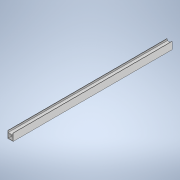
# Autodesk Inventor part: rail
Saved by Autodesk Inventor 2021 (Build 250183000, 183)
## iProperties
Created: 2021-04-01
Part Number: rail
Material: Generic
Document SubType Name: Modeling
Designer: miw14
Density: 1 g/cm^3
Appearance: Default
Mass: 103313 g
Surface Area: 104654 cm^2
Volume: 103313 cm^3
Author: miw14
Autodesk Inventor part; units mm, degrees
ref_plane "YZ Plane" through (0, 0, 0) normal (1, 0, 0) x (0, 1, 0)
ref_plane "XZ Plane" through (0, 0, 0) normal (0, 1, 0) x (-1, 0, 0)
ref_plane "XY Plane" through (0, 0, 0) normal (0, 0, 1) x (1, 0, 0)
sketch "Sketch1" plane through (0, 0, 0) normal (0, 0, 1) x (1, 0, 0)
  line L0 (85.725, -31.7513) -> (-85.725, -31.7513)
  line L1 (-85.725, -31.7513) -> (-85.725, 31.7513)
  line L2 (85.725, 31.7513) -> (85.725, -31.7513)
  line L3 (85.725, -31.7513) -> (-85.725, 31.7513) construction
  line L4 (-85.725, -31.7513) -> (85.725, 31.7513) construction
  line L5 (-85.725, 31.7513) -> (-98.425, 31.7513)
  line L6 (-98.425, 31.7513) -> (-98.425, -44.4487)
  line L7 (-98.425, -44.4487) -> (98.425, -44.4487)
  line L8 (98.425, -44.4487) -> (98.425, 31.7513)
  line L9 (98.425, 31.7513) -> (85.725, 31.7513)
  line L10 (-98.425, -44.4487) -> (98.425, -44.4487)
  line L11 (98.425, -44.4487) -> (98.425, -241.2987)
  line L12 (98.425, -241.2987) -> (-98.425, -241.2987)
  line L13 (-98.425, -241.2987) -> (-98.425, -44.4487)
  line L14 (-84.7979, -220.4745) -> (82.55, -220.4745)
  line L15 (82.55, -220.4745) -> (82.55, -65.6197)
  line L16 (82.55, -65.6197) -> (-84.7979, -65.6197)
  line L17 (-84.7979, -65.6197) -> (-84.7979, -220.4745)
  point P0 (0, 0)
  point P1 (98.425, -44.4487)
  dimension "d6" = 76.2
  dimension "d7" = 196.85
  dimension "d8" = 12.7
  dimension "d11" = 196.85
  dimension "d12" = 12.7
  constraints: 36 end point, 7 perpendicular, 5 parallel, 4 horizontal, 2 midpoint, 1 point on line
  measures "d6" distance of L7.end L8.end
  measures "d7" distance of L6.end L7.end
  measures "d8" distance of L8.end L2.start
  measures "d11" distance of L10.end L11.end
  measures "d12" distance of L1.end L5.end
extrude "Extrusion1" add sketch "Sketch1" along normal blind 6096
body "Solid1"
